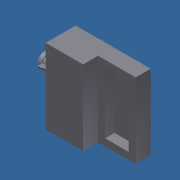
# Autodesk Inventor part: LEGO Brick 4488
Saved by Autodesk Inventor 2011 SP2 (Build 150309200, 309)
## iProperties
Created: 2011-09-28
Part Number: LEGO Brick 4488
Cost Center: 0 kg
Material: Steel
Document SubType Name: Modeling
Designer: BvH
Authority: 0 mm^3
Stock Number: =<Filenr>_<Document number>
Density: 7.85 g/cm^3
Company: Allseas Engineering BV
Subject: =<Title><TITLE 1_2> <TITLE 2_2>
Author: BvH
Act. Code: DW000
SaveDate: 2011-07-28
SaveTime: 18:32
FileName: Standard
TotalMass: 0 kg
TotalVolume: 0 mm^3
Autodesk Inventor part; units mm, degrees
ref_plane "YZ Plane" through (0, 0, 0) normal (1, 0, 0) x (0, 1, 0)
ref_plane "XZ Plane" through (0, 0, 0) normal (0, 1, 0) x (-1, 0, 0)
ref_plane "XY Plane" through (0, 0, 0) normal (0, 0, 1) x (1, 0, 0)
sketch "Sketch1" plane through (0, 0, 0) normal (0, 0, 1) x (1, 0, 0)
  line L0 (8, 1.6) -> (-8, 1.6)
  line L1 (-8, 1.6) -> (-8, -4.8)
  line L2 (-8, -4.8) -> (0, -4.8)
  line L3 (8, -1.6) -> (8, 1.6)
  line L4 (0, -4.8) -> (0, -1.6)
  line L5 (0, -1.6) -> (8, -1.6)
  line L6 (-11.2, 0) -> (11.2, 0) construction
  line L7 (0, -6.08) -> (0, 2.88) construction
  point P0 (0, 1.6)
  point P1 (8, 0)
  dimension "d0" = 16
  dimension "d1" = 3.2
  dimension "d2" = 6.4
  constraints: 12 end point, 3 point on line, 3 vertical, 2 horizontal, 2 midpoint
  measures "d0" distance between parallel lines of L3 L1
  measures "d1" distance between parallel lines of L5 L0
  measures "d2" distance between parallel lines of L0 L2
extrude "Extrusion1" add sketch "Sketch1" along normal mid plane 16
sketch "Sketch2" plane through (-8, 1.6, 8) normal (0, 1, 0) x (1, 0, 0)
  line L0 (4, 12) -> (12, 12) construction
  line L1 (12, 12) -> (12, 4) construction
  line L2 (12, 4) -> (4, 4) construction
  line L3 (4, 4) -> (4, 12) construction
  line L4 (-3.2, 8) -> (19.2, 8) construction
  line L5 (8, 19.2) -> (8, -3.2) construction
  circle A0 centre (4, 12) radius 2.5
  circle A1 centre (12, 12) radius 2.5
  circle A2 centre (12, 4) radius 2.5
  circle A3 centre (4, 4) radius 2.5
  point P0 (8, 12)
  point P1 (12, 8)
  dimension "d5" = 8
  dimension "d6" = 5
  constraints: 8 end point, 4 centre point, 4 coincident, 3 equal radius, 2 midpoint, 2 parallel, 2 perpendicular, 2 point on line, 1 horizontal
  measures "d5" distance between parallel lines of L1 L3
  measures "d6" diameter of A0
extrude "Extrusion2" add sketch "Sketch2" along normal blind 1.6
sketch "Sketch4" plane through (0, 0, 0) normal (0, 1, 0) x (-1, 0, 0)
  line L0 (8, -8) -> (8, 8) construction
  line L1 (14, 0) -> (7, 0) construction
  line L2 (8, 0) -> (8, -1.6)
  line L3 (8, -1.6) -> (9, -1.6)
  line L4 (9, -1.6) -> (9, -1.4)
  line L5 (9, -1.4) -> (12.2, -1.4)
  line L6 (12.2, -1.4) -> (12.2, -1.6)
  line L7 (12.2, -1.6) -> (13, -1.6)
  line L8 (13, -1.6) -> (13, 0)
  line L9 (13, 0) -> (8, 0)
  dimension "d9" = 2.8
  dimension "d11" = 3.2
  dimension "d12" = 5
  dimension "d13" = 3.2
  dimension "d14" = 0.8
  constraints: 16 end point, 4 horizontal, 4 vertical, 3 collinear
  measures "d9" diameter of L5 L9
  measures "d11" diameter of L7 L9
  measures "d12" distance between parallel lines of L8 L2
  measures "d13" distance of L4.end L5.end
  measures "d14" distance between parallel lines of L6 L8
revolve "Revolution1" add sketch "Sketch4" angle 360 about axis through (-13, 0, 0) along (1, 0, 0)
sketch "Sketch5" plane through (0, 0, 0) normal (0, 1, 0) x (-1, 0, 0)
  line L0 (9, 1.6) -> (9, -1.6) projected
  line L1 (8, -8) -> (8, 8) projected
  line L2 (9, -1.6) -> (8, -3.3321)
  line L3 (9, 1.6) -> (8, 3.3321)
  dimension "d16" = 30
  constraints: 4 end point, 2 point on line, 1 equal length
  measures "d16" angle of L3 L1
extrude "Extrusion3" add sketch "Sketch5" along normal mid plane 1.6
sketch "Sketch6" plane through (0, 0, 0) normal (0, 1, 0) x (-1, 0, 0)
  line L0 (13, 1.6) -> (13, -1.6) construction
  line L1 (13, -0.4) -> (10.9, -0.4)
  arc A0 (10.9, 0.4) -> (10.9, -0.4) centre (10.9, 0) ccw
  line L2 (10.9, 0.4) -> (13, 0.4)
  line L3 (13, 0.4) -> (13, -0.4)
  point P0 (13, 0)
  dimension "d19" = 0.8
  dimension "d20" = 2.5
  constraints: 6 end point, 2 horizontal, 2 midpoint, 2 point on circle, 2 tangent, 1 centre point, 1 vertical
  measures "d19" distance between parallel lines of L2 L1
extrude "Extrusion4" cut sketch "Sketch6" along normal through all both and the other way through all
sketch "Sketch7" plane through (0, -1.6, 8) normal (0, -1, 0) x (1, 0, 0)
  circle A0 centre (4, -4) radius 2.5 construction
  circle A1 centre (4, -12) radius 2.5 construction
  line L0 (1.5, -1.5) -> (6.5, -1.5)
  line L1 (6.5, -1.5) -> (6.5, -14.5)
  line L2 (6.5, -14.5) -> (1.5, -14.5)
  line L3 (1.5, -14.5) -> (1.5, -1.5)
  arc A2 (6.5, -5.783) -> (6.5, -10.217) centre (6.5, -8) ccw
  arc A3 (1.5, -10.217) -> (1.5, -5.783) centre (1.5, -8) ccw
  constraints: 8 end point, 6 tangent, 4 point on circle, 4 point on line, 2 centre point, 2 midpoint, 2 parallel, 1 horizontal, 1 perpendicular
extrude "Extrusion5" cut sketch "Sketch7" against normal blind 2
body "Solid1"
